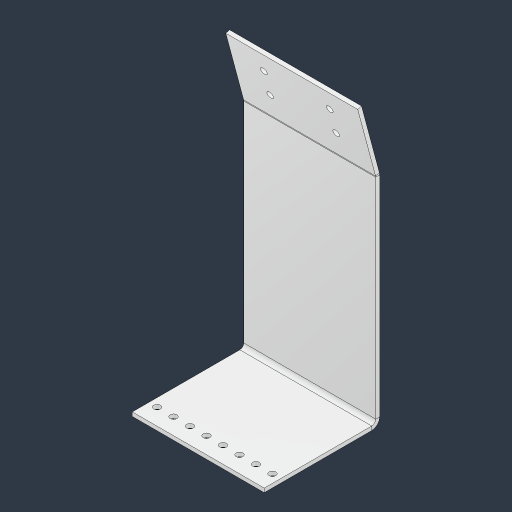
# Autodesk Inventor part: hopper_back_support
Saved by Autodesk Inventor 2024.3 (Build 283343000, 343)
## iProperties
Created: 2025-03-08
Part Number: hopper_back_support
Material: Aluminum 6061
Document SubType Name: Sheet Metal
Designer: marcu
Density: 2.7 g/cm^3
Sheet Metal Rule: Default
Appearance: Aluminum - Flat
Author: marcu
Autodesk Inventor part; units mm, degrees
ref_plane "YZ Plane" through (0, 0, 0) normal (1, 0, 0) x (0, 1, 0)
ref_plane "XZ Plane" through (0, 0, 0) normal (0, 1, 0) x (-1, 0, 0)
ref_plane "XY Plane" through (0, 0, 0) normal (0, 0, 1) x (1, 0, 0)
sketch "Sketch1" plane through (0, 0, 0) normal (0, 0, 1) x (1, 0, 0)
  line L0 (50.8, -84.1375) -> (-50.8, -84.1375)
  line L1 (-50.8, -84.1375) -> (-50.8, 84.1375)
  line L2 (-50.8, 84.1375) -> (50.8, 84.1375)
  line L3 (50.8, 84.1375) -> (50.8, -84.1375)
  line L4 (50.8, -84.1375) -> (-50.8, 84.1375) construction
  line L5 (-50.8, -84.1375) -> (50.8, 84.1375) construction
  point P0 (0, 0)
  dimension "d0" = 101.6
  dimension "d1" = 168.275
  measures "d0" distance of L1.end L2.end
  measures "d1" distance of L2.end L0.start
extrude "Plate1" add sketch "Sketch1" along normal blind 3.048
sketch "Sketch2" plane through (-50.8, 83.3486, 2.9441) normal (0, 0.258819, -0.9659258) x (-1, 0, 0)
  line L0 (-101.6, 0) -> (0, 0)
  line L1 (0, 0) -> (0, 53.975)
  line L2 (0, 53.975) -> (-101.6, 53.975)
  line L3 (-101.6, 53.975) -> (-101.6, 0)
  constraints: 6 end point, 1 horizontal, 1 perpendicular, 1 vertical
edge flange "Flange1" height 53.975 angle 15 thickness 3.048 bend radius 3.048 thickness toward (0, 0.258819, -0.9659258) relief straight relief width 3.048 relief depth 1.524 edges at (0, 84.1375, 3.048) wall of the first edge with corners at (50.8, 83.3486, 2.9441) (-50.8, 83.3486, 2.9441) (-50.8, 135.4845, 16.9139) (50.8, 135.4845, 16.9139)
bend "Bend1"
corner "Corner1"
sketch "Sketch3" plane through (50.8, 136.2733, 13.9698) normal (0, 0.258819, -0.9659258) x (-1, 0, 0)
  line L0 (0, -53.1724) -> (101.6, -53.1724) construction
  line L1 (101.6, 0) -> (101.6, -53.1724) construction
  line L2 (0, 0) -> (101.6, 0) construction
  line L3 (0, -53.1724) -> (0, 0) construction
  line L4 (25.4, -34.1224) -> (76.2, -34.1224) construction
  point P0 (50.8, -135.2456)
  point P1 (25.4, -15.0724)
  point P2 (76.2, -15.0724)
  point P3 (50.8, -34.1224)
  point P4 (50.8, 0)
  dimension "d15" = 50.8
  dimension "d18" = 19.05
  dimension "d21" = 19.05
  constraints: 2 end point, 2 horizontal, 2 midpoint, 1 vertical, 1 vertical alignment, 3 other
  measures "d15" distance of L4.start L4.end
  measures "d18" distance of L4.start point (25.4, -15.072)
  measures "d21" distance between parallel lines of L0 L4
hole "Hole1" at (25.4, 103.3136, 5.1382) at (-25.4, 103.3136, 5.1382) at (25.4, 121.7145, 10.0687) at (-25.4, 121.7145, 10.0687) direction (0, -0.258819, 0.9659258) diameter 5.1054 end through all clearance for "Flat Head Machine Screw (82)" size "#10" standard "Ansi Unified Screw Threads"
sketch "Sketch4" plane through (50.8, -81.0895, 0) normal (0, -1, 0) x (1, 0, 0)
  line L0 (-101.6, 0) -> (0, 0)
  line L1 (0, 0) -> (0, 88.9)
  line L2 (0, 88.9) -> (-101.6, 88.9)
  line L3 (-101.6, 88.9) -> (-101.6, 0)
  constraints: 6 end point, 1 horizontal, 1 perpendicular, 1 vertical
edge flange "Flange2" height 88.9 angle 90 thickness 3.048 bend radius 3.048 thickness toward (0, -1, 0) relief straight relief width 3.048 relief depth 1.524 edges at (0, -84.1375, 3.048) wall of the first edge with corners at (-50.8, -81.0895, 0) (50.8, -81.0895, 0) (50.8, -81.0895, 88.9) (-50.8, -81.0895, 88.9)
bend "Bend2"
corner "Corner2"
sketch "Sketch5" plane through (-50.8, -81.0895, 88.9) normal (0, 1, 0) x (1, 0, 0)
  line L0 (101.6, 82.804) -> (0, 82.804) construction
  line L1 (0, 82.804) -> (0, 0) construction
  line L2 (0, 0) -> (101.6, 0) construction
  line L3 (101.6, 82.804) -> (101.6, 0) construction
  line L4 (50.8, 0) -> (50.8, 12.7) construction
  line L5 (50.8, 12.7) -> (44.45, 12.7) construction
  point P0 (50.8, 88.9)
  point P1 (31.75, 12.7)
  point P2 (19.05, 12.7)
  point P3 (6.35, 12.7)
  point P4 (57.15, 12.7)
  point P5 (69.85, 12.7)
  point P6 (82.55, 12.7)
  point P7 (95.25, 12.7)
  dimension "d39" = 12.7
  dimension "d40" = 6.35
  dimension "d43" = 12.7
  constraints: 4 end point, 4 symmetric about line, 2 horizontal, 1 coincident, 1 midpoint, 1 vertical, 3 other
  measures "d39" distance of L4.start L4.end
  measures "d40" distance of L4.end L5.end
  measures "d43" distance of point (44.45, 12.7) point (31.75, 12.7)
hole "Hole2" at (-6.35, -81.0895, 76.2) at (-19.05, -81.0895, 76.2) at (-31.75, -81.0895, 76.2) at (-44.45, -81.0895, 76.2) at (44.45, -81.0895, 76.2) at (31.75, -81.0895, 76.2) at (19.05, -81.0895, 76.2) at (6.35, -81.0895, 76.2) direction (0, -1, 0) diameter 5.1054 end through all clearance for "Flat Head Machine Screw (82)" size "#10" standard "Ansi Unified Screw Threads"
equation "\"d27\" = Thickness"
equation "\"d2\" = Thickness"
equation "\"d3\" = BendReliefWidth"
equation "\"d4\" = BendReliefDepth"
equation "\"d5\" = MinimumRemnant"
equation "\"d6\" = TransitionRadius"
equation "\"d9\" = BendRadius"
equation "\"d10\" = CornerReliefSize"
equation "\"d11\" = GapSize"
equation "\"d12\" = JacobiRadiusSize"
equation "\"d29\" = BendReliefWidth"
equation "\"d30\" = BendReliefDepth"
equation "\"d31\" = MinimumRemnant"
equation "\"d32\" = TransitionRadius"
equation "\"d35\" = BendRadius"
equation "\"d36\" = CornerReliefSize"
equation "\"d37\" = GapSize"
equation "\"d38\" = JacobiRadiusSize"
equation "\"BendRadius\" = Thickness"
equation "\"BendReliefWidth\" = Thickness"
equation "\"BendReliefDepth\" = 0.5 * Thickness"
equation "\"CornerReliefSize\" = 4 * Thickness"
equation "\"MinimumRemnant\" = 2 * Thickness"
equation "\"TransitionRadius\" = BendRadius"
equation "\"JacobiRadiusSize\" = BendRadius"
equation "\"GapSize\" = Thickness"
equation "\"Thickness\" = 3.048"
body "Solid1"
